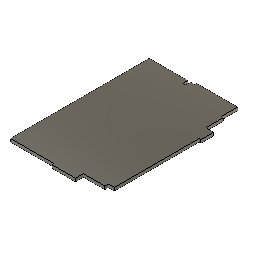
MAKPACbottom (Autodesk Fusion 360 design; units mm, degrees)
Autodesk Fusion 360 part; units mm, degrees
sketch "bottomSketch" plane through (0, 0, 0) normal (0, 0, 1) x (1, 0, 0) in component "bottom"
  line L0 (77, 139) -> (0, 139)
  line L1 (189, 50) -> (189, -120)
  line L2 (-192.8001, 143) -> (192.8001, -143) construction
  line L3 (91, 139) -> (91, 143)
  line L4 (0, 143) -> (0, -143) construction
  line L5 (192.8001, 143) -> (-192.8001, -143) construction
  line L6 (-192.8001, 143) -> (-192.8001, -143) construction
  line L7 (0, -139) -> (0, 139)
  line L8 (-192.8001, -143) -> (192.8001, -143) construction
  line L9 (192.8001, 143) -> (-192.8001, 143) construction
  line L10 (177.0001, 75) -> (192.8001, 75)
  line L11 (87.5001, -143) -> (87.5001, -139)
  line L12 (83, 139) -> (91, 139)
  line L13 (192.8001, 50) -> (189, 50)
  line L14 (192.8001, 75) -> (192.8001, 50)
  line L15 (177.0001, -120) -> (177.0001, -127)
  line L16 (173, 143) -> (173.0001, 110)
  line L17 (134.0001, -143) -> (87.5001, -143)
  line L18 (189, -120) -> (177.0001, -120)
  line L19 (83, 129) -> (83, 139)
  line L20 (177.0001, 110) -> (177.0001, 75)
  line L21 (173.0001, 110) -> (177.0001, 110)
  line L22 (77, 129) -> (83, 129)
  line L23 (134.0001, -127) -> (134.0001, -143)
  line L24 (77, 139) -> (77, 129)
  line L25 (91, 143) -> (173, 143)
  line L26 (192.8001, -143) -> (192.8001, 143) construction
  line L27 (87.5001, -139) -> (0, -139)
  line L28 (177.0001, -127) -> (134.0001, -127)
  dimension "d14" = 4
  dimension "d15" = 16
  dimension "d16" = 7
  constraint coincident L7.start L4
  constraint perpendicular L4 L27
  constraint coincident L0.end L4
  constraint perpendicular L0 L4
  constraint horizontal L9
  constraint vertical L6
  constraint horizontal L8
  constraint vertical L26
  measures "d14" distance of L11.end L11.start
  measures "d15" distance of L23.start L17.start
  measures "d16" distance of L15.end L15.start
extrude "Extrude2" add sketch "bottomSketch" along normal blind 6 in component "bottom"
component "bottom" placed x (1, 0, 0) y (0, 1, 0) z (0, 0, 1) at (0, 0, 0)
named bodies: "bottomBody"
